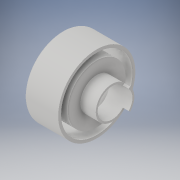
# Autodesk Inventor part: RearWheelRight
Saved by Autodesk Inventor 2017 (Build 210142000, 142)
## iProperties
Created: 2017-08-21
Part Number: RearWheelRight
Material: Generic
Document SubType Name: Modeling
Designer: MineV
Density: 1 g/cm^3
Appearance: Default
Author: MineV
Autodesk Inventor part; units mm, degrees
ref_plane "XZ Plane" through (0, 0, 0) normal (0, 1, 0) x (-1, 0, 0)
ref_plane "XY Plane" through (0, 0, 0) normal (0, 0, 1) x (1, 0, 0)
ref_plane "Work Plane1" through (20, 0, 0) normal (1, 0, 0) x (0, 1, 0)
sketch "Sketch7" plane through (0, 0, 0) normal (1, 0, 0) x (0, 1, 0)
  circle A0 centre (0, 0) radius 7.5
  circle A1 centre (0, 0) radius 20
  dimension "d28" = 15
  dimension "d29" = 40
  constraints: 2 centre point, 2 coincident
  measures "d28" diameter of A0
  measures "d29" diameter of A1
extrude "Wheel" add sketch "Sketch7" along normal blind 18
sketch "Sketch8" plane through (0, 0, 0) normal (1, 0, 0) x (0, 1, 0)
  circle A0 centre (0, 0) radius 13.5
  dimension "d33" = 27
  constraints: 1 centre point
  measures "d33" diameter of A0
extrude "Extrusion7" cut sketch "Sketch8" along normal blind 17
fillet "Fillet1" radius 2 1 edges at (0, -20, 0)
fillet "Fillet2" radius 1 1 edges at (0, -13.5, 0)
shell "Shell1" thickness 1.5 removed faces 1 at (18, 15.6396, -1.5954)
sketch "Sketch10" plane through (18, 0, 0) normal (1, 0, 0) x (0, 0, -1)
  circle A0 centre (0, 0) radius 8.5
  circle A1 centre (0, 0) radius 7.5 projected
  dimension "d41" = 17
  constraints: 1 centre point, 1 coincident
  measures "d41" diameter of A0
extrude "Extrusion9" add sketch "Sketch10" along normal blind 8
sketch "Sketch12" plane through (26, 0, 0) normal (1, 0, 0) x (0, 0, -1)
  circle A0 centre (0, 0) radius 8.5 projected
  circle A1 centre (0, 0) radius 7.5 projected
  line L0 (0, 0) -> (5.5902, -5)
  line L1 (0, 0) -> (5.5902, 5)
  circle A2 centre (0, 0) radius 7.5 projected
  line L2 (5.5902, 5) -> (5.5902, -5) construction
  line L3 (0, 0) -> (0, 5.0755) construction
  line L4 (5.5902, -5) -> (6.3355, -5.6667)
  line L5 (5.5902, 5) -> (6.3355, 5.6667)
  arc A3 (5.5902, -5) -> (5.5902, 5) centre (0, 0) ccw
  arc A4 (6.3355, -5.6667) -> (6.3355, 5.6667) centre (0, 0) ccw
  dimension "d53" = 10
  constraints: 12 end point, 8 point on circle, 2 centre point, 1 parallel, 1 vertical
  measures "d53" distance of L1.end L0.end
extrude "Extrusion11" add sketch "Sketch12" along normal blind 3 contours A0 L4 A1 L5 picked at (8.0097, 1.2845)
body "Solid1"
